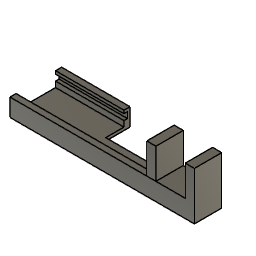
SensorMount (Autodesk Fusion 360 design; units mm, degrees)
Autodesk Fusion 360 part; units mm, degrees
sketch "Sketch1" plane through (0, 0, 0) normal (0, 0, 1) x (1, 0, 0)
  line L0 (-22.5, -8.5) -> (22.5, -8.5)
  line L1 (22.5, -8.5) -> (22.5, 8.5)
  line L2 (22.5, 8.5) -> (-22.5, 8.5)
  line L3 (-22.5, 8.5) -> (-22.5, -8.5)
  line L4 (-22.5, -8.5) -> (22.5, 8.5) construction
  line L5 (22.5, -8.5) -> (-22.5, 8.5) construction
  dimension "d3" = 17
  dimension "d5" = 45
  constraint horizontal L0
  constraint perpendicular L0 L1
  constraint parallel L0 L2
  constraint parallel L1 L3
  constraint coincident L4 origin
  constraint coincident L5 origin
  measures "d3" distance of L0.start L2.end
  measures "d5" distance of L1.end L2.end
extrude "Extrude1" add sketch "Sketch1" along normal blind 5.8
sketch "Sketch2" plane through (22.5, 0, 0) normal (1, 0, 0) x (0, 1, 0)
  line L0 (-8.5, 0) -> (8.5, 0)
  line L1 (8.5, 0) -> (8.5, 5.8)
  line L2 (8.5, 5.8) -> (-8.5, 5.8)
  line L3 (-8.5, 5.8) -> (-8.5, 0)
  line L4 (-7.65, 4.8) -> (7.65, 4.8)
  line L5 (7.65, 4.8) -> (7.65, 2.85)
  line L6 (7.65, 2.85) -> (-7.65, 2.85)
  line L7 (-7.65, 2.85) -> (-7.65, 4.8)
  line L8 (-7.65, 4.8) -> (7.65, 2.85) construction
  line L9 (7.65, 4.8) -> (-7.65, 2.85) construction
  line L10 (6.1, 4.8) -> (-6.2, 4.8)
  line L11 (-6.5, 5.8) -> (6.5, 5.8)
  line L12 (6.5, 5.8) -> (6.5, 1)
  line L13 (6.5, 1) -> (-6.5, 1)
  line L14 (-6.5, 1) -> (-6.5, 5.8)
  point P0 (0, 3.825)
  dimension "d9" = 15.3
  dimension "d10" = 1.95
  dimension "d11" = 0.85
  dimension "d17" = 1
  dimension "d18" = 1
  dimension "d20" = 2
  dimension "d21" = 2
  constraint horizontal L4
  constraint perpendicular L4 L5
  constraint parallel L4 L6
  constraint parallel L5 L7
  constraint coincident L8 P0
  constraint coincident L9 P0
  constraint coincident L4 L10.end
  constraint coincident L4 L10.start
  constraint horizontal L11
  constraint vertical L12
  constraint horizontal L13
  constraint vertical L14
  constraint coincident L2 L11.start
  measures "d9" distance of L5.end L6.end
  measures "d10" distance of L4.start L6.end
  measures "d11" distance of L3 L7
  measures "d17" distance of L2 L10
  measures "d18" distance of L0 L13
  measures "d20" distance of L3 L14
  measures "d21" distance of L1 L12
extrude "Extrude2" cut sketch "Sketch2" against normal up to surface (45 mm away) contours L2 L4 L10 L11 L12 L14 | L4 L6 L7 L14 | L4 L6 L10 L12 L14 | L4 L5 L6 L12 | L6 L12 L13 L14
sketch "Sketch3" plane through (22.5, 0, 0) normal (1, 0, 0) x (0, 1, 0)
  line L0 (6.5, 5.8) -> (6.5, 4.8)
  line L1 (6.5, 4.8) -> (7.65, 4.8)
  line L2 (7.65, 4.8) -> (7.65, 2.85)
  line L3 (7.65, 2.85) -> (6.5, 2.85)
  line L4 (6.5, 2.85) -> (6.5, 1)
  line L5 (6.5, 1) -> (-6.5, 1)
  line L6 (-6.5, 1) -> (-6.5, 2.85)
  line L7 (-6.5, 2.85) -> (-7.65, 2.85)
  line L8 (-7.65, 2.85) -> (-7.65, 4.8)
  line L9 (-7.65, 4.8) -> (-6.5, 4.8)
  line L10 (-6.5, 4.8) -> (-6.5, 5.8)
  line L11 (-6.5, 5.8) -> (-8.5, 5.8)
  line L12 (-8.5, 5.8) -> (-8.5, 0)
  line L13 (-8.5, 0) -> (8.5, 0)
  line L14 (8.5, 0) -> (8.5, 5.8)
  line L15 (8.5, 5.8) -> (6.5, 5.8)
  line L16 (-8.5, 5.8) -> (8.5, 5.8)
  line L17 (8.5, 5.8) -> (8.5, 0)
  line L18 (8.5, 0) -> (-8.5, 0)
  line L19 (-8.5, 0) -> (-8.5, 5.8)
  constraint horizontal L16
  constraint vertical L17
  constraint horizontal L18
  constraint vertical L19
  constraint coincident L13.end L14.start
  constraint coincident L11.end L12.start
extrude "Extrude3" add sketch "Sketch3" along normal blind 15.65
sketch "Sketch4" plane through (0, 0, 5.8) normal (0, 0, 1) x (-1, 0, 0)
  line L0 (-22.5, 6.5) -> (22.5, 6.5)
  line L1 (22.5, 6.5) -> (22.5, 8.5)
  line L2 (22.5, 8.5) -> (-38.15, 8.5)
  line L3 (-38.15, 8.5) -> (-38.15, -8.5)
  line L4 (-38.15, -8.5) -> (22.5, -8.5)
  line L5 (22.5, -8.5) -> (22.5, -6.5)
  line L6 (22.5, -6.5) -> (-22.5, -6.5)
  line L7 (-22.5, -6.5) -> (-22.5, 6.5)
  line L8 (-22.5, -6.5) -> (-22.5, -8.5)
  line L9 (-25.5, -8.5) -> (-25.5, 8.5)
  line L10 (-22.5, 6.5) -> (-22.5, -6.5)
  line L11 (-22.5, 6.5) -> (-22.5, 8.5)
  line L12 (-22.5, 8.5) -> (-25.5, 8.5)
  line L13 (-22.5, -8.5) -> (-25.5, -8.5)
  line L14 (-38.15, 8.5) -> (-35.15, 8.5)
  line L15 (-35.15, 8.5) -> (-35.15, -8.5)
  line L16 (-35.15, -8.5) -> (-38.15, -8.5)
  line L17 (-38.15, -8.5) -> (-38.15, 8.5)
  dimension "d24" = 3
  dimension "d25" = 3
  constraint coincident L6.end L7.start
  constraint coincident L4 L8.end
  constraint perpendicular L4 L8
  constraint coincident L4 L9.start
  constraint coincident L2 L9.end
  constraint perpendicular L2 L9
  constraint coincident L0.start L7.end
  constraint coincident L2 L11.end
  constraint perpendicular L2 L11
  constraint horizontal L14
  constraint vertical L15
  constraint horizontal L16
  constraint vertical L17
  constraint coincident L4 L15.end
  constraint coincident L2.end L3.start
  measures "d24" distance of L8.end L9.start
  measures "d25" distance of L15.end L3.end
extrude "Extrude4" add sketch "Sketch4" along normal blind 10 contours L2 L4 L7 L8 L9 L10 L11 L12 L13 | L2 L3 L4 L14 L15 L16 L17
sketch "Sketch5" plane through (0, 8.5, 0) normal (0, 1, 0) x (-1, 0, 0)
  line L0 (-38.15, 0) -> (22.5, 0)
  line L1 (22.5, 0) -> (22.5, 5.8)
  line L2 (22.5, 5.8) -> (-22.5, 5.8)
  line L3 (-22.5, 5.8) -> (-25.5, 5.8)
  line L4 (-25.5, 5.8) -> (-35.15, 5.8)
  line L5 (-35.15, 5.8) -> (-35.15, 15.8)
  line L6 (-35.15, 15.8) -> (-38.15, 15.8)
  line L7 (-38.15, 15.8) -> (-38.15, 0)
  line L8 (-38.15, 15.8) -> (0, 15.8)
  line L9 (0, 15.8) -> (0, 0)
  line L10 (0, 0) -> (-38.15, 0)
  line L11 (-38.15, 0) -> (-38.15, 15.8)
  constraint horizontal L8
  constraint vertical L9
  constraint horizontal L10
  constraint vertical L11
  constraint coincident L9.end L10.start
  constraint coincident L6.end L7.start
extrude "Extrude5" cut sketch "Sketch5" against normal blind 8 contours L0 L2 L3 L4 L5 L6 L7 L8 L9 L10 L11 | L2 L3 L4 L5 L8 L9
equation "Width = 15 mm"
equation "Height = 1.8 mm"
equation "d3 = Width + 2 mm"
equation "adjustableLength = 45 mm"
equation "d5 = adjustableLength"
equation "d6 = Height + 4 mm"
equation "Tol = 0.15 mm"
equation "d9 = Width + Tol * 2"
equation "d10 = Height + Tol"
equation "d11 = 1 mm - Tol"
equation "d22 = 15.5 mm + Tol"
